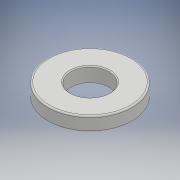
# Autodesk Inventor part: bearingWheel
Saved by Autodesk Inventor 2018.2 (Build 222227000, 227)
## iProperties
Created: 2018-02-27
Part Number: bearingWheel
Material: Generic
Document SubType Name: Modeling
Designer: mzhang
Density: 1 g/cm^3
Appearance: Default
Author: mzhang
Autodesk Inventor part; units mm, degrees
ref_plane "YZ Plane" through (0, 0, 0) normal (1, 0, 0) x (0, 1, 0)
ref_plane "XZ Plane" through (0, 0, 0) normal (0, 1, 0) x (-1, 0, 0)
ref_plane "XY Plane" through (0, 0, 0) normal (0, 0, 1) x (1, 0, 0)
sketch "Sketch1" plane through (0, 0, 0) normal (0, 0, 1) x (1, 0, 0)
  circle A0 centre (0, 0) radius 5.05
  circle A1 centre (0, 0) radius 11.05
  circle A2 centre (0, 0) radius 9.05
  circle A3 centre (0, 0) radius 7.05
  dimension "d0" = 10.1
  dimension "d1" = 6
  dimension "d2" = 2
  dimension "d3" = 2
  constraints: 4 centre point, 1 coincident
  measures "d0" diameter of A0
  measures "d1" radial gap between concentric circles of A0 A1
  measures "d2" radial gap between concentric circles of A1 A2
  measures "d3" radial gap between concentric circles of A0 A3
extrude "Extrusion1" add sketch "Sketch1" along normal blind 3.8 contours A1 | A2 | A3
fillet "Fillet1" radius 0.4 2 edges at (-11.05, 0, 3.8) (-11.05, 0, 0)
chamfer "Chamfer1" distance 0.25 angle 45 1 edges at (-5.05, 0, 3.8)
body "Solid1"
